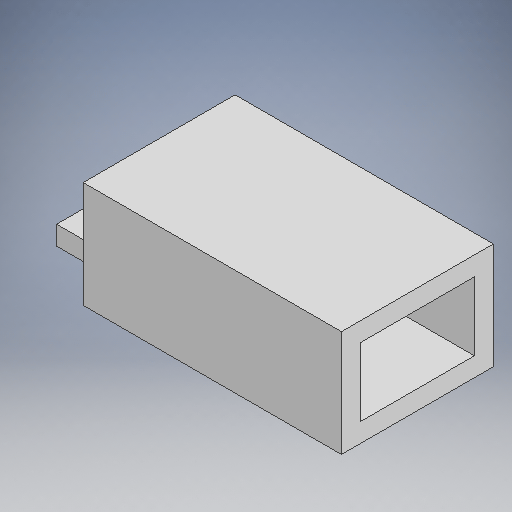
# Autodesk Inventor part: camsera_case_new_top
Saved by Autodesk Inventor 2025.2 (Build 292293000, 293)
## iProperties
Created: 2025-03-10
Part Number: camsera_case_new_top
Material: 일반
Document SubType Name: Modeling
Designer: jbhma
Density: 1 g/cm^3
Appearance: 기본값
Author: jbhma
Autodesk Inventor part; units mm, degrees
ref_plane "YZ Plane" through (0, 0, 0) normal (1, 0, 0) x (0, 1, 0)
ref_plane "XZ Plane" through (0, 0, 0) normal (0, 1, 0) x (-1, 0, 0)
ref_plane "XY Plane" through (0, 0, 0) normal (0, 0, 1) x (1, 0, 0)
sketch "스케치12" plane through (0, 0, 0) normal (0, 1, 0) x (-1, 0, 0)
  line L0 (0, 0) -> (-63, 0)
  line L1 (-63, 0) -> (-63, -30)
  line L2 (-63, -30) -> (0, -30)
  line L3 (0, -30) -> (0, 0)
  dimension "d57" = 63
  dimension "d58" = 30
  constraints: 8 end point, 2 parallel, 1 horizontal, 1 perpendicular
  measures "d57" distance of L2.end L1.end
  measures "d58" distance of L1.end L0.end
sketch "스케치22" plane through (0, 0, 0) normal (0, 1, 0) x (-1, 0, 0)
  line L0 (0, 0) -> (-63, 0)
  line L1 (-63, 0) -> (-63, 5)
  line L2 (-63, 5) -> (0, 5)
  line L3 (0, 5) -> (0, 0)
  line L4 (0, 5) -> (5, 5)
  line L5 (5, 5) -> (5, -35)
  line L6 (5, -35) -> (0, -35)
  line L7 (0, -35) -> (0, 5)
  line L8 (0, -35) -> (-63, -35)
  line L9 (-63, -35) -> (-63, -30)
  line L10 (-63, -30) -> (0, -30)
  line L11 (0, -30) -> (0, -35)
  dimension "d95" = 63
  dimension "d96" = 5
  dimension "d97" = 5
  constraints: 24 end point, 6 parallel, 3 horizontal, 3 perpendicular
  measures "d95" distance of L1.end L2.end
  measures "d96" distance of L0.end L1.end
  measures "d97" distance of L5.end L6.end
extrude "돌출16" add sketch "스케치22" along normal blind 28
extrude "돌출17" add sketch "스케치12" along normal blind 5
sketch "스케치23" plane through (0, 28, 0) normal (1, 0, 0) x (0, 0, -1)
  line L0 (0, 0) -> (30, 0)
  line L1 (30, 0) -> (30, -5)
  line L2 (30, -5) -> (0, -5)
  line L3 (0, -5) -> (0, 0)
  point P0 (0, -28)
  constraints: 8 end point, 2 parallel, 1 horizontal, 1 perpendicular
extrude "돌출18" add sketch "스케치23" along normal blind 63
sketch "스케치24" plane through (-5, 0, -35) normal (-1, 0, 0) x (0, 0, 1)
  point P0 (35, 0)
sketch "스케치25" plane through (-5, 0, -35) normal (-1, 0, 0) x (0, 0, 1)
  line L0 (30, 0) -> (10, 0)
  line L1 (10, 0) -> (10, 5)
  line L2 (10, 5) -> (30, 5)
  line L3 (30, 5) -> (30, 0)
  point P0 (35, 0)
  constraints: 8 end point, 2 parallel, 1 horizontal, 1 perpendicular
extrude "돌출19" add sketch "스케치25" along normal blind 17
sketch "스케치26" plane through (-5, 5, -5) normal (0, 1, 0) x (1, 0, 0)
  circle A0 centre (-8.5, 10) radius 3.5
  line L0 (-17, 0) -> (-17, 20) projected
  line L1 (0, 20) -> (-17, 20) projected
  point P0 (5, -5)
  dimension "d106" = 7
  dimension "d107" = 8.5
  dimension "d108" = 10
  constraints: 1 centre point
  measures "d106" diameter of A0
  measures "d107" distance from line of A0.centre L0
  measures "d108" distance from line of A0.centre L1
extrude "돌출20" cut sketch "스케치26" against normal blind 17
